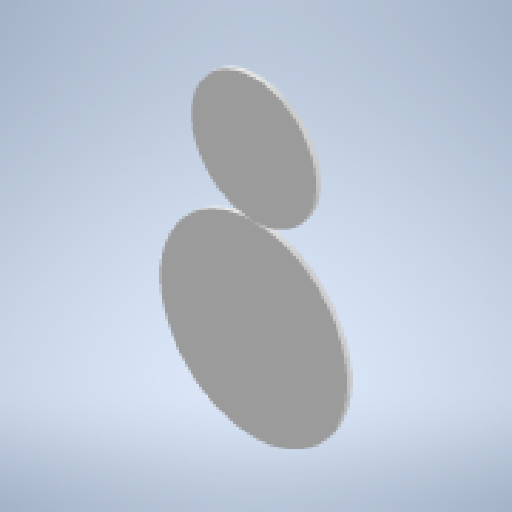
# Autodesk Inventor part: GearsTest
Saved by Autodesk Inventor 2023 (Build 270158030, 158C)
## iProperties
Created: 2024-09-26
Part Number: GearsTest
Material: Generic
Document SubType Name: Modeling
Designer: lvrectanus0
Density: 1 g/cm^3
Appearance: Default
Author: lvrectanus0
Autodesk Inventor part; units mm, degrees
ref_plane "YZ Plane" through (0, 0, 0) normal (1, 0, 0) x (0, 1, 0)
ref_plane "XZ Plane" through (0, 0, 0) normal (0, 1, 0) x (-1, 0, 0)
sketch "Sketch1" plane through (0, 0, 0) normal (0, 0, 1) x (1, 0, 0)
  circle A0 centre (0, 0) radius 14.351 projected
  circle A1 centre (0, 0) radius 82.55 projected
  circle A2 centre (0, 0) radius 21.59
  circle A3 centre (0, -51.435) radius 29.845
  circle A4 centre (0, 0) radius 81.28
  point P0 (0, -21.59)
  dimension "d0" = 162.56
  dimension "d1" = 43.18
  constraints: 3 centre point, 2 coincident, 2 tangent
  measures "d0" diameter of A4
  measures "d1" diameter of A2
ref_plane "Work Plane1" through (-15.4305, -15.4305, 1.524) normal (0, 0, 1) x (1, 0, 0)
extrude "Extrusion1" add sketch "Sketch1" along normal up to surface (1.524 mm away) contours A0 | A2
body "Solid1"
